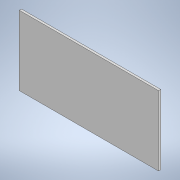
# Autodesk Inventor part: Rampe
Saved by Autodesk Inventor 2020.3 (Build 243373000, 373)
## iProperties
Created: 2020-09-30
Part Number: Rampe
Material: Generic
Document SubType Name: Modeling
Designer: Mara
Density: 1 g/cm^3
Appearance: Default
Author: Mara
Autodesk Inventor part; units mm, degrees
ref_plane "YZ Plane" through (0, 0, 0) normal (1, 0, 0) x (0, 1, 0)
ref_plane "XZ Plane" through (0, 0, 0) normal (0, 1, 0) x (-1, 0, 0)
ref_plane "XY Plane" through (0, 0, 0) normal (0, 0, 1) x (1, 0, 0)
sketch "Sketch1" plane through (0, 0, 0) normal (0, 0, 1) x (1, 0, 0)
  line L0 (-640, -320) -> (640, -320)
  line L1 (640, -320) -> (640, 320)
  line L2 (640, 320) -> (-640, 320)
  line L3 (-640, 320) -> (-640, -320)
  line L4 (-640, -320) -> (640, 320) construction
  line L5 (640, -320) -> (-640, 320) construction
  point P0 (0, 0)
  dimension "d0" = 1280
  dimension "d1" = 640
  constraints: 12 end point, 2 midpoint, 2 parallel, 1 horizontal, 1 perpendicular
  measures "d0" distance of L2.end L1.end
  measures "d1" distance of L1.end L0.end
extrude "Extrusion1" add sketch "Sketch1" along normal blind 20
body "Solid1"
